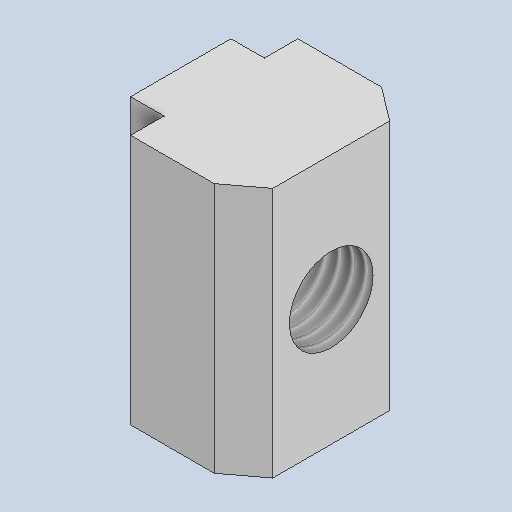
# Autodesk Inventor part: drazka
Saved by Autodesk Inventor 2025 (Build 290162000, 162)
## iProperties
Created: 2025-09-03
Part Number: drazka
Material: Generic
Document SubType Name: Modeling
Designer: Pravoslav
Density: 1 g/cm^3
Appearance: Default
Author: Pravoslav
Autodesk Inventor part; units mm, degrees
ref_plane "YZ Plane" through (0, 0, 0) normal (1, 0, 0) x (0, 1, 0)
ref_plane "XZ Plane" through (0, 0, 0) normal (0, 1, 0) x (-1, 0, 0)
ref_plane "XY Plane" through (0, 0, 0) normal (0, 0, 1) x (1, 0, 0)
sketch "Sketch1" plane through (0, 0, 0) normal (0, 1, 0) x (-1, 0, 0)
  line L0 (3.5, 5) -> (-3.5, 5)
  line L1 (-3.5, 5) -> (-3.5, -5)
  line L2 (-3.5, -5) -> (3.5, -5)
  line L3 (3.5, -5) -> (3.5, 5)
  line L4 (3.5, 5) -> (-3.5, -5) construction
  line L5 (-3.5, 5) -> (3.5, -5) construction
  line L6 (-1.5, 5) -> (-3.5, 3.5)
  line L7 (-1.5, -5) -> (-3.5, -3.5)
  line L8 (5.5, 3) -> (1.5, 3)
  line L9 (1.5, 3) -> (1.5, -3)
  line L10 (1.5, -3) -> (5.5, -3)
  line L11 (5.5, -3) -> (5.5, 3)
  line L12 (5.5, 3) -> (1.5, -3) construction
  line L13 (1.5, 3) -> (5.5, -3) construction
  point P0 (0, 0)
  point P1 (-3.5, 0)
  point P2 (3.5, 0)
  point P3 (3.5, 3)
  point P4 (3.5, -3)
  dimension "d0" = 7
  dimension "d1" = 10
  dimension "d2" = 5
  dimension "d3" = 5
  dimension "d4" = 3.5
  dimension "d5" = 3.5
  dimension "d6" = 4
  dimension "d7" = 6
  constraints: 28 end point, 6 midpoint, 4 parallel, 4 point on line, 2 horizontal, 2 perpendicular
  measures "d0" distance of L2.end L1.end
  measures "d1" distance of L1.end L0.end
  measures "d2" distance from line of L3 L6.start
  measures "d3" distance from line of L3 L7.start
  measures "d4" distance of point (-3.5, 0) L7.end
  measures "d5" distance of point (-3.5, 0) L6.end
  measures "d6" distance of L10.end L9.end
  measures "d7" distance of L9.end L8.end
extrude "Extrusion1" add sketch "Sketch1" along normal blind 15 contours L3 L8 L9 L10 L2 L7 L1 L6 L0 | L8 L11 L10 L3 | L3 L10 L9 L8
sketch "Sketch2" plane through (-5.5, 0, -3) normal (-1, 0, 0) x (0, 0, 1)
  circle A0 centre (3, 7.5) radius 2.5
  line L0 (0, 0) -> (6, 0) projected
  line L1 (0, 0) -> (0, 15) projected
  point P0 (3, 0)
  dimension "d10" = 5
  dimension "d11" = 7.5
  dimension "d12" = 3
  constraints: 1 centre point
  measures "d10" diameter of A0
  measures "d11" distance from line of L0 A0.centre
  measures "d12" distance from line of L1 A0.centre
extrude "Extrusion2" cut sketch "Sketch2" against normal through all
thread "Thread1" size "M5x0.8" class "6H" standard "ISO Metric profile" full length
body "Solid1"
